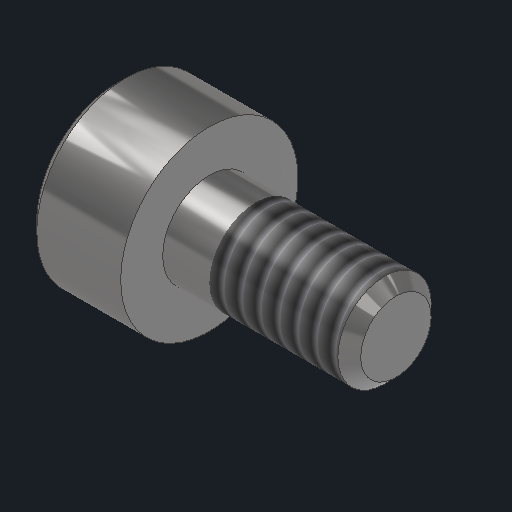
# Autodesk Inventor part: CB2-4
Saved by Autodesk Inventor 2022 (Build 260153000, 153)
## iProperties
Category: PARTsolutions
Company: MISUMI
Created: 2017-11-08
Part Number: CB2-4
Catalog Web Link: www.cadenas.de
Description: 在庫有
Vendor: MISUMI
Document SubType Name: Modeling
Designer: psAdmin
Manufacturer: MISUMI
Mass: 0.257303 g
Surface Area: 0.745169 cm^2
Volume: 0.0327775 cm^3
Density: 7.85 g/cm^3
Material: 鋼、炭素鋼
Appearance: 半つや出し
PSOL_IDENT_0: {$CADENAS_DATA\23d-libs\misumi\metric\27_screws_nuts\cb_fa.prj},149 {VTYP=3D},{NB=CB2-4},{LINA=CB2-4
PSOL_IDENT_1: },{NN=CB},{DATE=24.04.2017 09:49:34},{GEOMDATE=17.02.2014 00:00:00},{VERSION=},{LINEID=10},{LINESUBI
PSOL_IDENT_2: D=-1},{WBVAR=L}  {NB=CB2-4},{LINA=CB2-4},{KT=DUMMY},{PN=CB2-4},{MAT=4137 Steel},{HARD=38~43HRC},{ST=
PSOL_IDENT_3: Black Oxide},{M=2},{L=4},{LL=Full Thread},{L1=60},{TYPE=CB},{M1=2.000},{L0=4,5,6,8,10,12,15},{NDM=2}
PSOL_IDENT_4: ,{KDM=1.508532},{MP=2x0.4},{P=0.4},{A=3.8},{E=2.0},{B=1.5},{V=0.2}
NN: CB
NT: Hexagon Socket Head Cap Screws
NB: CB2-4
NBSYN: $PN.
LINA: CB2-4
PN: CB2-4
MAT: 4137 Steel
HARD: 38~43HRC
ST: Black Oxide
M: 2
L: 4
LL: Full Thread
MP: 2x0.4
A: 3.8
E: 2.0
B: 1.5
SUPPLIER: MISUMI
ARTICLENO: CB2-4
BOMINFO: CB2-4
CREATOR: CADENAS GmbH
購入先: ミスミ
在庫数: 0.0
Title: CB2-4
Author: Cadenas PARTsolutions
Comments: Hexagon Socket Head Cap Screws
Autodesk Inventor part; units mm, degrees
sketch "Sketch_1" plane through (0, 0, 0) normal (0, 0, 1) x (1, 0, 0)
  line L0 (4, 0) -> (-2, 0)
  line L1 (-2, 0) -> (-2, 1.7)
  line L2 (-2, 1.7) -> (-1.8, 1.9)
  line L3 (-1.8, 1.9) -> (0, 1.9)
  line L4 (0, 1.9) -> (0, 1)
  line L5 (0, 1) -> (3.7545, 1)
  line L6 (3.7545, 1) -> (4, 0.7545)
  line L7 (4, 0.7545) -> (4, 0)
  line L8 (4, 0) -> (-2, 0)
  constraints: 18 end point
revolve "Revolution1" add sketch "Sketch_1" angle 360 about axis through (4, 0, 0) along (1, 0, 0)
thread "Thread1" size "M2x0.4" class "6g" standard "ISO Metric profile" length 2.7545
sketch "Sketch_4_ALT_Drilling_1" plane through (0, 0, 0) normal (0, 0, 1) x (1, 0, 0)
  line L0 (-0.799, 0) -> (-2, 0)
  line L1 (-2, 0) -> (-2, 0.75)
  line L2 (-2, 0.75) -> (-1, 0.75)
  line L3 (-1, 0.75) -> (-0.799, 0)
  line L4 (-0.799, 0) -> (-2, 0)
  constraints: 10 end point
revolve "Revolution2" cut sketch "Sketch_4_ALT_Drilling_1" angle 360 about axis through (-0.799, 0, 0) along (1, 0, 0)
sketch "Sketch_3" plane through (-2, 0, 0) normal (1, 0, 0) x (0, 0, -1)
  line L0 (-0.75, -0.433) -> (0, -0.866)
  line L1 (0, -0.866) -> (0.75, -0.433)
  line L2 (0.75, -0.433) -> (0.75, 0.433)
  line L3 (0.75, 0.433) -> (0, 0.866)
  line L4 (0, 0.866) -> (-0.75, 0.433)
  line L5 (-0.75, 0.433) -> (-0.75, -0.433)
  constraints: 12 end point
extrude "Extrusion1" cut sketch "Sketch_3" along normal blind 1
ref_plane "bolt_to_nut_XY" through (4, 0, 0) normal (1, 0, 0) x (0, 0, -1)
ref_plane "bolt_to_nut_YZ" through (4, 0, 0) normal (0, 0, -1) x (0, 1, 0)
ref_plane "bolt_to_nut_ZX" through (4, 0, 0) normal (0, 1, 0) x (1, 0, 0)
ref_plane "screw1_XY" through (0, 0, 0) normal (1, 0, 0) x (0, 0, -1)
ref_plane "screw1_YZ" through (0, 0, 0) normal (0, 0, -1) x (0, 1, 0)
ref_plane "screw1_ZX" through (0, 0, 0) normal (0, 1, 0) x (1, 0, 0)
body "Solid1"
